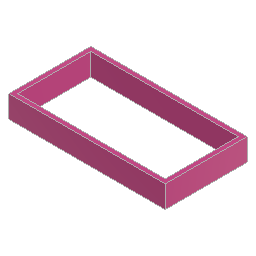
Tweezer-Holdster (Autodesk Fusion 360 design; units mm, degrees)
Autodesk Fusion 360 part; units mm, degrees
sketch "Sketch1" plane through (0, 0, 3.175) normal (0, 0, 1) x (-1, 0, 0)
  line L0 (0, 0) -> (0, 297.942)
  line L1 (0, 297.942) -> (-407.924, 297.942)
  line L2 (-407.924, 297.942) -> (-407.924, 0)
  line L3 (-407.924, 0) -> (0, 0)
  line L4 (0, 192.942) -> (-105, 192.942)
  line L5 (-105, 192.942) -> (-105, 137.942)
  line L6 (-105, 137.942) -> (0, 137.942)
  line L7 (0, 137.942) -> (0, 192.942)
  line L8 (-2.95, 189.992) -> (-102.05, 189.992)
  line L9 (-102.05, 189.992) -> (-102.05, 140.892)
  line L10 (-102.05, 140.892) -> (-2.95, 140.892)
  line L11 (-2.95, 140.892) -> (-2.95, 189.992)
  point P0 (0, 192.942)
  dimension "d168" = 105
  dimension "d169" = 55
  constraint horizontal L4
  constraint vertical L5
  constraint horizontal L6
  constraint vertical L7
  constraint coincident P0 L4.start
  measures "d168" distance of P0 L4.end
  measures "d169" distance of P0 L6.end
extrude "Extrude1" add sketch "Sketch1" along normal blind 15 contours L0 L4 L5 L6 L7
equation "d168 = TweezerCarrierWidth"
equation "d169 = TweezerCarrierLength"
equation "d170 = -HoldersterWallWidth + SmallTolerence"
equation "d171 = HoldersterHeightLow"
equation "SmallTolerence = 0.05 mm"
equation "HoldersterWallWidth = 3 mm"
equation "HoldersterHeightLow = 15 mm"
equation "TweezerCarrierWidth = 105 mm"
equation "TweezerCarrierLength = 55 mm"
